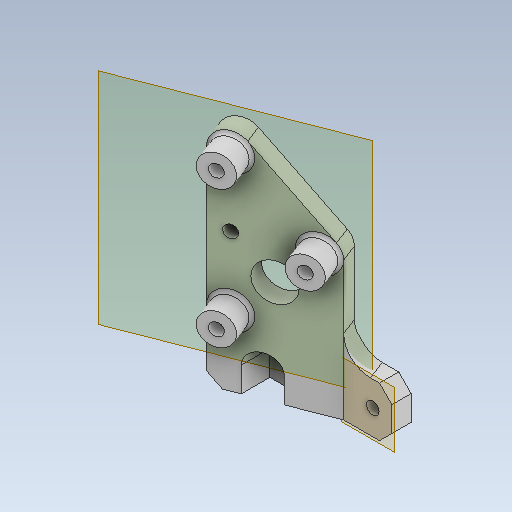
# Autodesk Inventor part: jc_conn_1
Saved by Autodesk Inventor 2020 (Build 240168000, 168)
## iProperties
Created: 2021-02-18
Part Number: jc_conn_1
Material: Generic
Document SubType Name: Modeling
Designer: Shuang Peng
Density: 1 g/cm^3
Appearance: Default
Author: Shuang Peng
Autodesk Inventor part; units mm, degrees
ref_plane "YZ Plane" through (0, 0, 0) normal (1, 0, 0) x (0, 1, 0)
ref_plane "XZ Plane" through (0, 0, 0) normal (0, 1, 0) x (-1, 0, 0)
ref_plane "XY Plane" through (0, 0, 0) normal (0, 0, 1) x (1, 0, 0)
ref_plane "Work Plane1" through (-20.789463, 15.2, 8.150078) normal (-0.3618889, 0, -0.9322212) x (-0.9322212, 0, 0.3618889)
sketch "Sketch2" plane through (-20.789463, 15.2, 8.150078) normal (-0.3618889, 0, -0.9322212) x (-0.9322212, 0, 0.3618889)
  circle A0 centre (-11, 0) radius 1
  circle A1 centre (0, 11) radius 1
  circle A2 centre (0, -11) radius 1
  circle A3 centre (-11, 0) radius 3
  circle A4 centre (0, 11) radius 3
  circle A5 centre (0, -11) radius 3
  line L0 (0, 11) -> (3, 11)
  line L1 (0, -11) -> (3, -11)
  line L2 (3, -11) -> (3, 11)
  line L3 (0, 11) -> (-2.12132, 13.12132)
  line L4 (-2.12132, 13.12132) -> (-13.12132, 2.12132)
  line L5 (-13.12132, 2.12132) -> (-11, 0)
  line L6 (3, -11) -> (3, -14)
  line L7 (3, -14) -> (-14, -14)
  line L8 (-14, -14) -> (-14, 0)
  point P0 (-22.329802, -15.2)
  dimension "d6" = 6
  dimension "d4" = 6
  dimension "d5" = 6
  dimension "d7" = 3
  constraints: 18 end point, 4 point on circle, 3 coincident, 3 parallel, 2 centre point, 2 perpendicular, 1 collinear, 1 horizontal, 1 horizontal alignment, 1 tangent, 2 other
  measures "d4" diameter of A3
  measures "d5" diameter of A4
  measures "d7" distance of L1.end L6.end
extrude "Extrusion1" add sketch "Sketch2" along normal blind 3 contours A0 | L0 L3 A1 | L0 A4 L3 A1 | A1 L3 L0 | A1 L3 A4 L0 | L2 A5 L7 L8 A3 L4 A4 | A5 | L6 L7 A5 | A3 | A2
sketch "Sketch4" plane through (-23.586127, 1.2, 9.235745) normal (0, -1, 0) x (0.9322212, 0, -0.3618889)
  line L0 (25.995086, -3.034057) -> (28.45793, -2.856683)
  line L1 (27.32334, 0.069374) -> (28.45793, -2.856683)
  line L2 (27.32334, 0.069374) -> (25.329802, -0.0742)
  line L3 (25.329802, -0.0742) -> (6.556451, -7.362027)
  line L4 (6.556451, -7.362027) -> (-4.022207, -15.90347)
  line L5 (-2.883579, -18.83994) -> (-4.022207, -15.90347)
  line L6 (-2.883579, -18.83994) -> (8.077612, -9.989632)
  line L7 (8.077612, -9.989632) -> (25.995086, -3.034057)
  line L8 (17, 0) -> (0, 0)
  line L9 (0, 0) -> (0, -3)
  line L10 (17, -3) -> (0, -3)
  line L11 (17, 0) -> (17, -3)
  line L12 (6.556451, -7.362027) -> (6.556451, 0)
  line L13 (17, 0) -> (0, 0)
  line L14 (25.329802, -0.0742) -> (24.244135, 2.722464)
  line L15 (24.244135, 2.722464) -> (17.231103, 0)
  line L16 (17, 0) -> (17, -3)
  line L17 (17, 0) -> (17.231103, 0)
  point P0 (6.556451, 0)
  dimension "d11" = 3
  constraints: 8 end point, 3 perpendicular, 2 point on line, 1 parallel
  measures "d11" distance of L2.end L14.end
ref_plane "Work Plane2" through (-35.564286, -7, -23.748518) normal (0, -1, 0) x (0.7068322, 0, -0.7073813)
extrude "Extrusion2" add sketch "Sketch4" along normal up to surface (8.2 mm away) contours L3 L12 L10 L11 L17 L15 L14 | L12 L8 L11 L10
sketch "Sketch5" plane through (-23.586127, 1.2, 9.235745) normal (0, 1, 0) x (0.9322212, 0, -0.3618889)
  line L0 (17, 0) -> (17, 3)
  line L1 (17.231103, 0) -> (17, 0)
  line L2 (24.244135, -2.722464) -> (17.231103, 0)
  line L3 (25.329802, 0.0742) -> (24.244135, -2.722464)
  line L4 (6.556451, 7.362027) -> (25.329802, 0.0742)
  line L5 (6.556451, 3) -> (6.556451, 7.362027)
  line L6 (17, 3) -> (6.556451, 3)
  line L7 (24.244135, -2.722464) -> (17.231103, 0)
  line L8 (24.244135, -2.722464) -> (24.213869, -2.800429)
  line L9 (24.213869, -2.800429) -> (17, 0)
  point P0 (25.329802, 0.0742)
  constraints: 4 end point, 1 parallel, 1 perpendicular
extrude "Extrusion3" add sketch "Sketch5" against normal up to surface (8.2 mm away) contours L1 L2 L8 L9
sketch "Sketch6" plane through (-24.671794, 1.2, 6.439081) normal (0, -1, 0) x (0.9322212, 0, -0.3618889)
  line L0 (6.556451, 0) -> (6.556451, 3)
  line L1 (6.556451, 3) -> (0, 3)
  line L2 (0, 3) -> (0, 0)
  line L3 (6.556451, 0) -> (0, 0)
  line L4 (6.556451, -4.362027) -> (6.556451, 3)
  line L5 (6.556451, 0) -> (0, 0)
  line L6 (6.556451, 0) -> (6.556451, -4.362027)
  line L7 (0, 0) -> (6.556451, -4.362027)
  point P0 (25.329802, 2.9258)
  constraints: 2 end point
extrude "Extrusion4" add sketch "Sketch6" along normal up to surface (8.2 mm away)
sketch "Sketch7" plane through (0, -7, 0) normal (0, 0, -1) x (-1, 0, 0)
  circle A0 centre (3.06915, 4) radius 1.6
  circle A1 centre (17.06915, 4) radius 1.6
  circle A2 centre (3.06915, 4) radius 1.6
  line L0 (20.1383, 8) -> (0, 8)
  line L1 (20.1383, 8) -> (20.1383, 0)
  line L2 (0, 0) -> (20.1383, 0)
  line L3 (0, 8) -> (0, 0)
  circle A3 centre (3.06915, 4) radius 1
  circle A4 centre (17.06915, 4) radius 1
  point P0 (0, 7)
  dimension "d21" = 2
  dimension "d22" = 2
  constraints: 2 centre point, 2 coincident
  measures "d21" diameter of A3
  measures "d22" diameter of A4
extrude "Extrusion5" cut sketch "Sketch7" against normal blind 10 contours A3 | A4
ref_plane "Work Plane3" through (-7.738366, 1.2, 3.083634) normal (0, 0, 1) x (1, 0, 0)
sketch "Sketch8" plane through (-7.738366, 1.2, 3.083634) normal (0, 0, 1) x (1, 0, 0)
  circle A0 centre (-9.330784, -4.2) radius 1
  line L0 (-9.330784, -4.2) -> (-9.330784, -11.2) construction
  line L1 (-11.830784, -4.2) -> (-11.830784, -11.2)
  line L2 (-6.830784, -11.2) -> (-6.830784, -4.2)
  arc A1 (-6.830784, -4.2) -> (-11.830784, -4.2) centre (-9.330784, -4.2) ccw
  arc A2 (-11.830784, -11.2) -> (-6.830784, -11.2) centre (-9.330784, -11.2) ccw
  point P0 (7.738366, -1.2)
  point P1 (-9.330784, -7.7)
  dimension "d26" = 7
  dimension "d27" = 5
  constraints: 8 end point, 4 point on circle, 4 tangent, 2 centre point, 1 midpoint, 1 parallel, 1 vertical
  measures "d26" distance of L0.start L0.end
  measures "d27" diameter of A2
extrude "Extrusion6" cut sketch "Sketch8" along normal blind 10
sketch "Sketch9" plane through (-21.87513, 15.2, 5.353415) normal (-0.3618889, 0, -0.9322212) x (-0.9322212, 0, 0.3618889)
  circle A0 centre (-11, 0) radius 1 projected
  circle A1 centre (0, 11) radius 1 projected
  circle A2 centre (0, -11) radius 1 projected
  circle A3 centre (0, -11) radius 1
  circle A4 centre (-11, 0) radius 1
  circle A5 centre (0, 11) radius 1
  point P0 (-22.329802, -15.2)
  dimension "d30" = 2
  dimension "d31" = 2
  dimension "d32" = 2
  constraints: 3 centre point, 3 coincident
  measures "d30" diameter of A3
  measures "d31" diameter of A4
  measures "d32" diameter of A5
extrude "Extrusion7" cut sketch "Sketch9" against normal blind 10
thicken "Thicken1" operation add thickness 0.2 both sides no extend neighbours yes toward (0, -1, 0) faces at (-17.878042, 1.2, 2.242017)
fillet "Fillet1" radius 4 1 edges at (-8.2812, 1, 1.6853)
chamfer "Chamfer2" distance 2 angle 45 3 edges at (0, -7, 1.5418) (0, 1, 1.5418) (-24.129, -7, 7.8374)
fillet "Fillet2" radius 1 1 edges at (-16.3783, 1, 3.2195)
sketch "Sketch10" plane through (-21.87513, 15.2, 5.353415) normal (-0.3618889, 0, -0.9322212) x (-0.9322212, 0, 0.3618889)
  circle A0 centre (0, 0) radius 1.5 projected
  circle A1 centre (0, 0) radius 1
  point P0 (-22.329802, -15.2)
  dimension "d45" = 2
  constraints: 1 centre point, 1 coincident
  measures "d45" diameter of A1
extrude "Extrusion8" cut sketch "Sketch10" against normal blind 10 contours A1
sketch "Sketch11" plane through (-21.87513, 15.2, 5.353415) normal (-0.3618889, 0, -0.9322212) x (-0.9322212, 0, 0.3618889)
  circle A0 centre (0, 0) radius 1
  circle A1 centre (0, -11) radius 1
  circle A2 centre (0, 11) radius 1
  circle A3 centre (-11, 0) radius 1
  line L0 (3, -13.2) -> (-14.792978, -13.2)
  line L1 (3, -13.2) -> (3, 11)
  arc A4 (3, 11) -> (-2.12132, 13.12132) centre (0, 11) ccw
  line L2 (-2.12132, 13.12132) -> (-13.12132, 2.12132)
  arc A5 (-13.12132, 2.12132) -> (-14, 0) centre (-11, 0) ccw
  line L3 (-14, 0) -> (-14, -10.2)
  arc A6 (-14.792978, -12.590609) -> (-14, -10.2) centre (-18, -10.2) ccw
  line L4 (-14.792978, -12.590609) -> (-14.792978, -13.2)
  circle A7 centre (0, -11) radius 1
  line L5 (0, -11) -> (-11, 0)
  circle A8 centre (-5.5, -5.5) radius 3
  point P0 (-22.329802, -15.2)
  dimension "d48" = 6
  constraints: 2 end point, 1 centre point, 1 midpoint
  measures "d48" diameter of A8
extrude "Extrusion9" cut sketch "Sketch11" against normal blind 10 contours A8 L5 | L5 A8
sketch "Sketch12" plane through (-20.789463, 15.2, 8.150078) normal (0.3618889, 0, 0.9322212) x (0.9322212, 0, -0.3618889)
  circle A0 centre (5.5, -5.5) radius 3
  circle A1 centre (0, 0) radius 1
  line L0 (-1, -22.2) -> (-3, -20.2)
  line L1 (-1, -22.2) -> (1.309038, -22.2)
  line L2 (1.309038, -22.2) -> (1.309038, -18.2)
  ellipse E0 centre (3.990805, -18.2) end of major axis (6.672572, -18.2) minor radius 2.5 (6.672572, -18.2) -> (1.309038, -18.2) ccw
  line L3 (6.672572, -18.2) -> (6.672572, -22.2)
  line L4 (6.672572, -22.2) -> (14, -22.2)
  line L5 (14, -10.2) -> (14, -22.2)
  line L6 (14, 0) -> (14, -10.2)
  arc A2 (14, 0) -> (13.12132, 2.12132) centre (11, 0) ccw
  line L7 (2.12132, 13.12132) -> (13.12132, 2.12132)
  arc A3 (2.12132, 13.12132) -> (-3, 11) centre (0, 11) ccw
  line L8 (-3, 11) -> (-3, -20.2)
  circle A4 centre (11, 0) radius 1
  circle A5 centre (0, 11) radius 1
  circle A6 centre (0, -11) radius 1
  circle A7 centre (0, -11) radius 2.5
  circle A8 centre (0, 11) radius 2.5
  circle A9 centre (11, 0) radius 2.5
  point P0 (22.329802, -15.2)
  dimension "d51" = 5
  dimension "d52" = 5
  dimension "d53" = 5
  constraints: 3 centre point, 3 coincident, 1 other
  measures "d51" diameter of A7
  measures "d52" diameter of A8
  measures "d53" diameter of A9
extrude "Extrusion10" add sketch "Sketch12" along normal blind 4 contours A7 | A8 | A9
fillet "Fillet3" radius 0.5 3 edges at (-12.8656, 15.2, 5.074) (-23.12, 26.2, 9.0548) (-23.12, 4.2, 9.0548)
body "Solid1"
